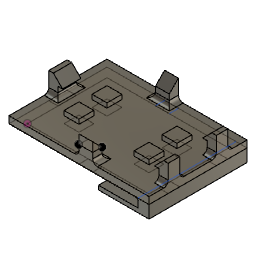
weather_station_battery_charger_IC v11 (Autodesk Fusion 360 design; units mm, degrees)
Autodesk Fusion 360 part; units mm, degrees
note: some values were not read from the file. Chosen so that the rebuilt part matches the saved one: which pieces of a blend or face edit are solid. Set by a fixed rule: which sketch regions a step uses.
sketch "Sketch1" plane through (0, 0, 0) normal (0, 0, 1) x (1, 0, 0)
  line L0 (0, 0) -> (26.5, 0)
  line L1 (26.5, 0) -> (26.5, 17.35)
  line L2 (26.5, 17.35) -> (0, 17.35)
  line L3 (0, 17.35) -> (0, 0)
  line L4 (-2, -2) -> (28.5, -2)
  line L5 (28.5, -2) -> (28.5, 19.35)
  line L6 (28.5, 19.35) -> (-2, 19.35)
  line L7 (-2, 19.35) -> (-2, -2)
  line L8 (-2, 6.675) -> (0, 6.675)
  line L9 (0, 6.675) -> (0, 10.675)
  line L10 (0, 10.675) -> (-2, 10.675)
  line L11 (-2, 10.675) -> (-2, 6.675)
  line L12 (13.25, -2) -> (16.25, -2)
  line L13 (16.25, -2) -> (16.25, 0)
  line L14 (16.25, 0) -> (13.25, 0)
  line L15 (13.25, 0) -> (13.25, -2)
  line L16 (10.5651, 17.35) -> (13.5651, 17.35)
  line L17 (13.5651, 17.35) -> (13.5651, 19.35)
  line L18 (13.5651, 19.35) -> (10.5651, 19.35)
  line L19 (10.5651, 19.35) -> (10.5651, 17.35)
  line L20 (26.5, 2.175) -> (28.5, 2.175)
  line L21 (28.5, 2.175) -> (28.5, 4.675)
  line L22 (28.5, 4.675) -> (26.5, 4.675)
  line L23 (26.5, 4.675) -> (26.5, 2.175)
  line L24 (26.5, 12.675) -> (28.5, 12.675)
  line L25 (28.5, 12.675) -> (28.5, 15.175)
  line L26 (28.5, 15.175) -> (26.5, 15.175)
  line L27 (26.5, 15.175) -> (26.5, 12.675)
  line L28 (4, 4) -> (7.25, 4)
  line L29 (7.25, 4) -> (7.25, 7.25)
  line L30 (7.25, 7.25) -> (4, 7.25)
  line L31 (4, 7.25) -> (4, 4)
  line L32 (22.5, 4) -> (19.25, 4)
  line L33 (19.25, 4) -> (19.25, 7.25)
  line L34 (19.25, 7.25) -> (22.5, 7.25)
  line L35 (22.5, 7.25) -> (22.5, 4)
  line L36 (4, 13.35) -> (7.25, 13.35)
  line L37 (7.25, 13.35) -> (7.25, 10.1)
  line L38 (7.25, 10.1) -> (4, 10.1)
  line L39 (4, 10.1) -> (4, 13.35)
  line L40 (19.25, 10.1) -> (22.5, 10.1)
  line L41 (22.5, 10.1) -> (22.5, 13.35)
  line L42 (22.5, 13.35) -> (19.25, 13.35)
  line L43 (19.25, 13.35) -> (19.25, 10.1)
  line L44 (26.1, -2) -> (26.1, 19.35)
  dimension "d1" = 26.5
  dimension "d2" = 17.35
  dimension "d3" = 2
  dimension "d4" = 2
  dimension "d5" = 2
  dimension "d6" = 2
  dimension "d7" = 4
  dimension "d8" = 6.675
  dimension "d9" = 3
  dimension "d10" = 3
  dimension "d11" = 2.5
  dimension "d12" = 2.5
  dimension "d13" = 8
  dimension "d14" = 2.175
  dimension "d15" = 4
  dimension "d16" = 4
  dimension "d17" = 3.25
  dimension "d18" = 3.25
  dimension "d19" = 3.25
  dimension "d20" = 3.25
  dimension "d21" = 4
  dimension "d22" = 4
  dimension "d23" = 3.25
  dimension "d24" = 3.25
  dimension "d25" = 4
  dimension "d26" = 4
  dimension "d27" = 3.25
  dimension "d28" = 3.25
  dimension "d29" = 4
  dimension "d30" = 4
  constraint horizontal L0
  constraint vertical L1
  constraint horizontal L2
  constraint vertical L3
  constraint coincident L0.start L3.end
  constraint horizontal L4
  constraint vertical L5
  constraint horizontal L6
  constraint vertical L7
  constraint horizontal L8
  constraint vertical L9
  constraint horizontal L10
  constraint vertical L11
  constraint coincident L3 L9.end
  constraint coincident L7 L8.start
  constraint horizontal L12
  constraint vertical L13
  constraint horizontal L14
  constraint vertical L15
  constraint coincident L0 L13.end
  constraint midpoint L4 L12.start
  constraint horizontal L16
  constraint vertical L17
  constraint horizontal L18
  constraint vertical L19
  constraint coincident L6 L17.end
  constraint coincident L2 L16.start
  constraint horizontal L20
  constraint vertical L21
  constraint horizontal L22
  constraint vertical L23
  constraint coincident L5 L21.end
  constraint coincident L1 L20.start
  constraint horizontal L24
  constraint vertical L25
  constraint horizontal L26
  constraint vertical L27
  constraint coincident L5 L25.end
  constraint coincident L1 L24.start
  constraint horizontal L28
  constraint vertical L29
  constraint horizontal L30
  constraint vertical L31
  constraint horizontal L32
  constraint vertical L33
  constraint horizontal L34
  constraint vertical L35
  constraint horizontal L36
  constraint vertical L37
  constraint horizontal L38
  constraint vertical L39
  constraint horizontal L40
  constraint vertical L41
  constraint horizontal L42
  constraint vertical L43
  constraint coincident L4 L44.start
  constraint coincident L6 L44.end
  constraint perpendicular L6 L44
  measures "d1" distance of L0.start L0.end
  measures "d2" distance of L0.start L2.end
  measures "d3" distance of L0.start L4
  measures "d4" distance of L2.end L6
  measures "d5" distance of L0.end L5
  measures "d7" distance of L8 L10
  measures "d8" distance of L2.end L10
  measures "d9" distance of L13 L15
  measures "d10" distance of L17 L19
  measures "d11" distance of L21.end L20
  measures "d12" distance of L24 L26
  measures "d13" distance of L22 L24.end
  measures "d14" distance of L0.end L20
  measures "d15" distance of L0 L28
  measures "d16" distance of L3 L31
  measures "d17" distance of L29.end L30.end
  measures "d18" distance of L28.end L29.end
  measures "d19" distance of L37.end L38.end
  measures "d20" distance of L36.start L38.end
  measures "d21" distance of L3 L39
  measures "d22" distance of L2 L36
  measures "d23" distance of L32.end L33.end
  measures "d24" distance of L33.end L34.end
  measures "d25" distance of L0 L32
  measures "d26" distance of L1 L35
  measures "d27" distance of L40.start L40.end
  measures "d28" distance of L40.start L42.end
  measures "d29" distance of L26.end L41
  measures "d30" distance of L2 L42
extrude "Extrude3" add sketch "Sketch1" along normal blind 3.7 contours L0 L4 L12 L13 L14 L15 | L3 L7 L8 L9 L10 L11 | L2 L6 L16 L17 L18 L19 | L1 L5 L20 L21 L22 L23 | L1 L5 L24 L25 L26 L27 makes body 1 at (26.5, 3.0083, 1.2333) makes body 2 at (14.25, 0, 1.2333) makes body 3 at (26.5, 13.5083, 1.2333) makes body 4 at (-2, 8.0083, 2.4667) makes body 5 at (12.5651, 19.35, 1.2333)
extrude "Extrude2" add sketch "Sketch1" along normal blind 1.5 contours L0 L2 L3 L9 L14 L16 L44 | L0 L3 L4 L7 L8 L15 | L0 L4 L13 L44 | L2 L3 L6 L7 L10 L19 | L0 L1 L2 L23 L27 L44 | L0 L1 L4 L5 L20 L44 | L1 L2 L5 L6 L26 L44 | L2 L6 L17 L44 | L1 L5 L22 L24 bodies 1 2 4 5 3
extrude "Extrude1" add sketch "Sketch1" along normal blind 2.5 contours L28 L29 L30 L31 | L32 L33 L34 L35 | L36 L37 L38 L39 | L40 L41 L42 L43 bodies 1
sketch "Sketch3" plane through (0, 0, 3.7) normal (0, 0, 1) x (-1, 0, 0)
  line L0 (2, -10.675) -> (2, -6.675)
  line L1 (2, -6.675) -> (0, -6.675)
  line L2 (0, -6.675) -> (0, -10.675)
  line L3 (0, -10.675) -> (2, -10.675)
  line L4 (2, -6.675) -> (-1, -6.675)
  line L5 (-1, -6.675) -> (-1, -10.675)
  line L6 (-1, -10.675) -> (2, -10.675)
  line L7 (2, -10.675) -> (2, -6.675)
  dimension "d37" = 3
  constraint horizontal L4
  constraint vertical L5
  constraint horizontal L6
  constraint vertical L7
  constraint coincident L0.end L1.start
  constraint coincident L0.start L3.end
  measures "d37" distance of L0.end L4.end
sketch "Sketch5" plane through (0, 0, 3.7) normal (0, 0, 1) x (-1, 0, 0)
  line L0 (-10.5651, -19.35) -> (-10.5651, -17.35)
  line L1 (-10.5651, -17.35) -> (-13.5651, -17.35)
  line L2 (-13.5651, -17.35) -> (-13.5651, -19.35)
  line L3 (-13.5651, -19.35) -> (-10.5651, -19.35)
  line L4 (-10.5651, -19.35) -> (-13.5651, -19.35)
  line L5 (-13.5651, -19.35) -> (-13.5651, -17.35)
  line L6 (-13.5651, -17.35) -> (-10.5651, -17.35)
  line L7 (-10.5651, -17.35) -> (-10.5651, -19.35)
  dimension "d39" = 2
  constraint horizontal L4
  constraint vertical L5
  constraint horizontal L6
  constraint vertical L7
  constraint coincident L0.start L3.end
  measures "d39" distance of L0.start L0.end
sketch "Sketch6" plane through (0, 0, 3.7) normal (0, 0, 1) x (-1, 0, 0)
  line L0 (-26.5, -15.175) -> (-26.5, -12.675)
  line L1 (-26.5, -12.675) -> (-28.5, -12.675)
  line L2 (-28.5, -12.675) -> (-28.5, -15.175)
  line L3 (-28.5, -15.175) -> (-26.5, -15.175)
  line L4 (-28.5, -15.175) -> (-25.5, -15.175)
  line L5 (-25.5, -15.175) -> (-25.5, -12.675)
  line L6 (-25.5, -12.675) -> (-28.5, -12.675)
  line L7 (-28.5, -12.675) -> (-28.5, -15.175)
  dimension "d41" = 3
  constraint horizontal L4
  constraint vertical L5
  constraint horizontal L6
  constraint vertical L7
  constraint coincident L2.end L3.start
  constraint coincident L1.end L2.start
  measures "d41" distance of L2.end L4.end
sketch "Sketch7" plane through (0, 0, 3.7) normal (0, 0, 1) x (-1, 0, 0)
  line L0 (-26.5, -4.675) -> (-26.5, -2.175)
  line L1 (-26.5, -2.175) -> (-28.5, -2.175)
  line L2 (-28.5, -2.175) -> (-28.5, -4.675)
  line L3 (-28.5, -4.675) -> (-26.5, -4.675)
  line L4 (-28.5, -2.175) -> (-25.5, -2.175)
  line L5 (-25.5, -2.175) -> (-25.5, -4.675)
  line L6 (-25.5, -4.675) -> (-28.5, -4.675)
  line L7 (-28.5, -4.675) -> (-28.5, -2.175)
  dimension "d43" = 3
  constraint horizontal L4
  constraint vertical L5
  constraint horizontal L6
  constraint vertical L7
  constraint coincident L1.end L2.start
  constraint coincident L2.end L3.start
  measures "d43" distance of L1.end L4.end
sketch "Sketch8" plane through (0, 0, 3.7) normal (0, 0, 1) x (-1, 0, 0)
  line L0 (-13.25, 0) -> (-13.25, 2)
  line L1 (-13.25, 2) -> (-16.25, 2)
  line L2 (-16.25, 2) -> (-16.25, 0)
  line L3 (-16.25, 0) -> (-13.25, 0)
  line L4 (-13.15, 2) -> (-16.25, 2)
  line L5 (-16.25, 2) -> (-16.25, 0)
  line L6 (-16.25, 0) -> (-13.25, 0)
  line L7 (-13.25, 0) -> (-13.25, 2)
  constraint horizontal L4
  constraint vertical L5
  constraint horizontal L6
  constraint vertical L7
  constraint coincident L0.end L1.start
  constraint coincident L2.end L3.start
extrude "Extrude4" add sketch "Sketch3" sketch "Sketch5" sketch "Sketch7" sketch "Sketch8" sketch "Sketch6" along normal blind 2 of sketch 2 of sketch 3 of sketch 4 of sketch 5 bodies 1
chamfer "Chamfer1" distance 2 angle 45 5 edges at (12.0651, 17.35, 5.7) (14.75, 0, 5.7) (25.5, 3.425, 5.7) (25.5, 13.925, 5.7) (1, 8.675, 5.7) on bodies 1
extrude "Extrude5" add sketch "Sketch1" against normal blind 1.85 contours L0 L1 L4 L5 L20 L44 | L1 L2 L5 L6 L26 L44 | L1 L5 L20 L21 L22 L23 | L1 L5 L22 L24 | L1 L5 L24 L25 L26 L27 bodies 1
sketch "Sketch9" plane through (0, 0, -1.85) normal (0, 0, -1) x (1, 0, 0)
  line L0 (28.5, -19.35) -> (28.5, 2)
  line L1 (28.5, 2) -> (26.1, 2)
  line L2 (26.5, 0) -> (26.5, -17.35)
  line L3 (26.1, -19.35) -> (28.5, -19.35)
  line L4 (28.5, 2) -> (17.5, 2)
  line L5 (17.5, 2) -> (17.5, -19.3454)
  line L6 (17.5, -19.3454) -> (28.5, -19.3454)
  line L7 (28.5, -19.3454) -> (28.5, 2)
  line L8 (26.1, 0) -> (26.5, 0)
  line L9 (26.5, -17.35) -> (26.1, -17.35)
  line L10 (26.1, 2) -> (26.1, 0)
  line L11 (26.1, -17.35) -> (26.1, -19.35)
  dimension "d55" = 11
  constraint horizontal L4
  constraint vertical L5
  constraint horizontal L6
  constraint vertical L7
  constraint coincident L0.end L1.start
  measures "d55" distance of L5.end L6.end
extrude "Extrude6" add sketch "Sketch9" along normal blind 0.9 contours L0 L1 L2 L4 L6 L7 L8 L9 L10 L11 | L2 L4 L5 L6 L8 L9 L10 L11 bodies 1
fillet "Fillet1" radius 1 15 edges at (27.5, 15.175, 1.5) (26.5, 13.925, 1.5) (27.5, 4.675, 1.5) (26.5, 3.425, 1.5) (10.5651, 18.35, 1.5) (14.75, 0, 1.5) (13.25, -1, 1.5) (-1, 10.675, 1.5) (-1, 6.675, 1.5) (27.5, 2.175, 1.5) (27.5, 12.675, 1.5) (12.0651, 17.35, 1.5) (13.5651, 18.35, 1.5) (0, 8.675, 1.5) (16.25, -1, 1.5) on bodies 1
fillet "Fillet2" radius 0.5 6 edges at (26.1, -1, -1.85) (26.1, 18.3477, -1.85) (26.5, 8.675, -1.85) (26.1, 18.35, 0) (26.1, -1, 0) (26.5, 8.675, 0) on bodies 1
delete_face "DeleteFace1" 1 faces at (25.5636, 13.2382, 1.502) on bodies 1
delete_face "DeleteFace2" 1 faces at (25.5636, 2.7382, 1.502) on bodies 1
equation "d4 = d3"
equation "d5 = d3"
equation "d6 = d3"
equation "d8 = ( d2 - d7 ) / 2"
equation "d10 = d9"
equation "d12 = d11"
equation "d14 = ( d2 - d13 - 2 * d11 ) / 2"
equation "d16 = d15"
equation "d18 = d17"
equation "d19 = d17"
equation "d20 = d17"
equation "d21 = d15"
equation "d22 = d15"
equation "d23 = d17"
equation "d24 = d17"
equation "d25 = d15"
equation "d26 = d15"
equation "d27 = d17"
equation "d28 = d17"
equation "d29 = d15"
equation "d30 = d15"
